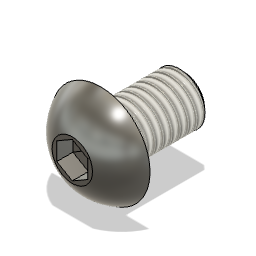
assembly (Autodesk Fusion 360 archive; units mm, degrees)
design "Broached Hexagon Socket Button Head Cap Screw ASME B18.3.4M - M5 x 0.8 x 8 Steel Grade 2 Plain"
description: Broached Hexagon Socket Button Head Cap Screw ASME B18.3.4M - M5 x 0.8 x 8
part number: BHSBHCS ASME B18.3.4M - M5 x 0.8 x 8 Steel Grade 2 Plain
Autodesk Fusion 360 part; units mm, degrees
sketch "Sketch1" plane through (0, 0, 0) normal (0, 1, 0) x (1, 0, 0)
  line L0 (-2.5, 0) -> (-2.5, 8)
  line L1 (-2.5, 8) -> (0, 8)
  line L2 (0, 8) -> (0, -2.75)
  line L3 (-2.5, 0) -> (-4.75, 0)
  line L4 (0, -2.75) -> (-1.95, -2.75)
  arc A0 (-4.75, 0) -> (-1.95, -2.75) centre (0, 2.0359) ccw
  dimension "d9" = 5
  dimension "d66" = 9.5
  dimension "d98" = 3.9
  dimension "d105" = 2.75
  dimension "d106" = 8
  constraint perpendicular L0 L1
  constraint perpendicular L0 L3
  constraint coincident origin L3
  constraint vertical L0
  constraint vertical L2
  constraint coincident origin L2
  constraint perpendicular L2 L4
  constraint coincident L2 A0.centre
  measures "d105" distance of L3 L4
  measures "d106" distance of origin L1
revolve "Revolve1" add sketch "Sketch1" angle 360 about axis through (0, 0, -8) along (0, 0, 1)
ref_plane "WorkPlane1" through (0, 0, 2.75) normal (0, 0, 1) x (1, 0, 0)
sketch "Sketch6" plane through (0, 0, 2.75) normal (0, 0, 1) x (1, 0, 0)
  line L0 (-1.5, 0) -> (1.5, 0) construction
  line L1 (0, 0) -> (-1.5, 0.866)
  line L2 (-1.5, -0.866) -> (-1.5, 0.866)
  line L3 (-1.5, -0.866) -> (0, 0)
  dimension "d91" = 150
  dimension "d107" = 3
  constraint horizontal L0
  constraint midpoint L1.start L0
  constraint coincident L1.start L3.end
  constraint perpendicular L0 L2
  constraint midpoint L0.start L2
  constraint coincident L1.end L2.end
  measures "d91" angle of L0 L1
  measures "d107" distance of L0.end L2
extrude "Extrude1" cut sketch "Sketch6" against normal blind 1.56
pattern_circular "C-Pattern1" count 6 over 360 about axis through (0, 0, 1.75) along (0, 0, 1) of "Extrude1"
extrude "Extrude2" cut 1 faces at (0, 0, 1.19) along direction (0, 0, -1) blind 1.56 draft -85
fillet "Fillet5" radius 0.2 1 edges at (-2.3308, 0.904, 0)
thread "Thread2" "ANSI Metric M Profile 5.0 M5x0.8 4g6g" major diameter 4.901 minor diameter 4.007 pitch 0.8 angle 60 resizes the face on face at (-2.4876, 0.2489, -5.4) from (0, 0, -1.6) to (0, 0, -8)
sketch "Sketch5" plane through (0, 0, 0) normal (0, 1, 0) x (1, 0, 0)
  line L0 (0, 8) -> (0, -2.75)
  line L1 (0, 8) -> (-2.55, 8)
  line L2 (-2.55, 8) -> (-2.55, 7.5092)
  line L3 (-2.55, 7.5092) -> (-2.0092, 8)
  dimension "d108" = 0.4908
  dimension "d109" = 2.0092
  dimension "d110" = 2.55
  constraint coincident L0.start L1.start
  constraint perpendicular L1 L2
  constraint coincident L1 L3.end
  measures "d108" distance of L1 L2.end
  measures "d109" distance of L0 L3.end
  measures "d110" distance of L0 L2
revolve "Revolve2" cut sketch "Sketch5" angle 360 about axis through (0, 0, -8) along (0, 0, 1)
equation "d9 = adsk_nomdia"
equation "adsk_nomlen = 8.00 mm"
equation "adsk_headh = 2.75 mm"
equation "adsk_headdia = 9.50 mm"
equation "adsk_nomdia = 5.00 mm"
equation "adsk_philwidth = 3.00 mm"
equation "d31 = -adsk_phildepth"
equation "adsk_phildepth = 1.56 mm"
equation "d66 = adsk_headdia"
equation "d71 = adsk_headh"
equation "d76 = -adsk_phildepth"
equation "adsk_thrlen = 6.40 mm"
equation "adsk_endpointdia = 4.01848 mm"
equation "adsk_startlen = 0.49076 mm"
equation "d96 = adsk_thrlen"
equation "d98 = adsk_philwidth * 1.3"
equation "adsk_midfillet = 0.20 mm"
equation "d104 = adsk_midfillet"
equation "d105 = adsk_headh"
equation "d106 = adsk_nomlen"
equation "d107 = adsk_philwidth"
equation "d108 = adsk_startlen"
equation "d109 = adsk_endpointdia / 2"
equation "d110 = adsk_nomdia * 0.51"

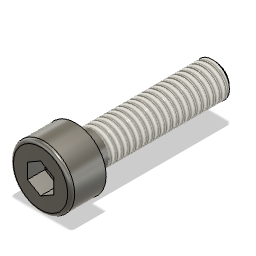
design "Broached Hexagon Socket Head Cap Screw ANSI B18.3.1M - M4x0.7 x 16 Steel Grade 2 Plain"
description: Broached Hexagon Socket Head Cap Screw ANSI B18.3.1M - M4x0.7 x 16
part number: BSHCS ANSI B18.3.1M - M4x0.7 x 16 Steel Grade 2 Plain
Autodesk Fusion 360 part; units mm, degrees
sketch "Sketch1" plane through (0, 0, 0) normal (0, 1, 0) x (1, 0, 0)
  line L0 (-2, 0) -> (-2, 16)
  line L1 (-2, 16) -> (0, 16)
  line L2 (0, 16) -> (0, -4)
  line L3 (-2, 0) -> (-3.5, 0)
  line L4 (-3.5, 0) -> (-3.5, -4)
  line L5 (-3.5, -4) -> (0, -4)
  dimension "d9" = 4
  dimension "d66" = 7
  dimension "d101" = 16
  dimension "d102" = 4
  constraint perpendicular L0 L1
  constraint collinear origin L1.end L2.end
  constraint perpendicular L0 L3
  constraint coincident origin L3
  constraint vertical L0
  constraint vertical L2
  constraint parallel L2 L4
  constraint coincident L2 L5.end
  constraint perpendicular L2 L5
  measures "d101" distance of origin L1
  measures "d102" distance of L3.end L5
revolve "Revolve1" add sketch "Sketch1" angle 360 about axis through (0, 0, -16) along (0, 0, 1)
ref_plane "WorkPlane1" through (0, 0, 4) normal (0, 0, 1) x (1, 0, 0)
sketch "Sketch6" plane through (0, 0, 4) normal (0, 0, 1) x (1, 0, 0)
  line L0 (-1.5, 0) -> (1.5, 0) construction
  line L1 (0, 0) -> (-1.5, 0.866)
  line L2 (-1.5, -0.866) -> (-1.5, 0.866)
  line L3 (-1.5, -0.866) -> (0, 0)
  dimension "d100" = 150
  dimension "d103" = 3
  constraint horizontal L0
  constraint midpoint L1.start L0
  constraint coincident L1.start L3.end
  constraint perpendicular L0 L2
  constraint midpoint L0.start L2
  constraint coincident L1.end L2.end
  measures "d100" angle of L0 L1
  measures "d103" distance of L0.end L2
extrude "Extrude1" cut sketch "Sketch6" against normal blind 2
pattern_circular "C-Pattern1" count 6 over 360 about axis through (0, 0, 1.75) along (0, 0, 1) of "Extrude1"
extrude "Extrude2" cut 1 faces at (0, -0.5774, 2) along direction (0, 0, -1) blind 2 draft -85
thread "Thread2" "ANSI Metric M Profile 4.0 M4x0.7 4g6g" major diameter 3.908 minor diameter 3.128 pitch 0.7 angle 60 resizes the face on face at (-1.9975, 0.0997, -5.3333) from (0, 0, -1.8294) to (0, 0, -16)
fillet "Fillet4" radius 0.4 1 edges at (-3.2631, 1.2657, 4)
sketch "Sketch7" plane through (0, 0, 0) normal (0, 1, 0) x (1, 0, 0)
  line L0 (-2.04, 16) -> (-2.04, 15.5706)
  line L1 (-2.04, 15.5706) -> (-1.5706, 16)
  line L2 (0, 16) -> (0, -4)
  line L3 (-2.04, 16) -> (0, 16)
  dimension "d104" = 1.5706
  dimension "d105" = 2.04
  dimension "d106" = 0.4294
  constraint coincident L2.start L3.end
  constraint perpendicular L2 L3
  constraint coincident L1.end L3
  constraint perpendicular L0 L3
  measures "d104" distance of L1.end L2
  measures "d105" distance of L0 L2.start
  measures "d106" distance of L0.end L3
revolve "Revolve3" cut sketch "Sketch7" angle 360 about axis through (0, 0, 1.75) along (0, 0, 1)
equation "d9 = adsk_nomdia"
equation "adsk_nomlen = 16.00 mm"
equation "adsk_headh = 4.00 mm"
equation "adsk_headdia = 7.00 mm"
equation "adsk_nomdia = 4.00 mm"
equation "adsk_philwidth = 3.00 mm"
equation "d31 = -adsk_phildepth"
equation "adsk_phildepth = 2.00 mm"
equation "d66 = adsk_headdia"
equation "d71 = adsk_headh"
equation "d76 = -adsk_phildepth"
equation "adsk_thrlen = 14.170585 mm"
equation "d84 = adsk_thrlen"
equation "d86 = adsk_nomdia * 0.1"
equation "adsk_startlen = 0.429415 mm"
equation "adsk_endpointdia = 3.14117 mm"
equation "d101 = adsk_nomlen"
equation "d102 = adsk_headh"
equation "d103 = adsk_philwidth"
equation "d104 = adsk_endpointdia / 2"
equation "d105 = adsk_nomdia * 0.51"
equation "d106 = adsk_startlen"
